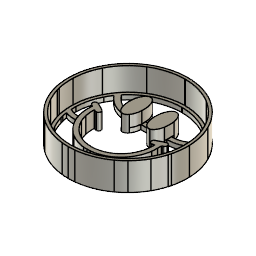
Smiley Face v5 (Autodesk Fusion 360 design; units mm, degrees)
Autodesk Fusion 360 part; units mm, degrees
(part 1 of 2)
sketch "Sketch4" plane through (0, 0, 0) normal (0, 0, 1) x (1, 0, 0)
  spline S0 degree 3 poles (22.3929, -49.7183) (18.1084, -49.2352) (14.0604, -47.6727) (10.6177, -45.1732) knots 0 0 0 0 1 1 1 1
  spline S1 degree 3 poles (10.6177, -45.1732) (9.3741, -44.2703) (8.777, -43.7559) (7.5724, -42.5496) knots 0 0 0 0 1 1 1 1
  spline S2 degree 3 poles (7.5724, -42.5496) (5.8834, -40.8584) (4.627, -39.2036) (3.4694, -37.1458) knots 0 0 0 0 1 1 1 1
  spline S3 degree 3 poles (3.4694, -37.1458) (2.6439, -35.6786) (1.7398, -33.529) (1.3502, -32.1074) knots 0 0 0 0 1 1 1 1
  spline S4 degree 3 poles (1.3502, -32.1074) (1.2509, -31.7452) (1.1157, -31.2562) (1.0497, -31.0207) knots 0 0 0 0 1 1 1 1
  spline S5 degree 3 poles (1.0497, -31.0207) (0.5782, -29.3376) (0.2735, -26.3861) (0.3562, -24.3029) knots 0 0 0 0 1 1 1 1
  spline S6 degree 3 poles (0.3562, -24.3029) (0.5048, -20.5588) (1.3013, -17.4096) (2.9297, -14.1273) knots 0 0 0 0 1 1 1 1
  spline S7 degree 3 poles (2.9297, -14.1273) (5.04, -9.8738) (7.9486, -6.665) (12.0751, -4.0377) knots 0 0 0 0 1 1 1 1
  spline S8 degree 3 poles (12.0751, -4.0377) (15.652, -1.7603) (20.598, -0.3264) (24.8627, -0.3305) knots 0 0 0 0 1 1 1 1
  spline S9 degree 3 poles (35.9401, -2.8345) (38.3777, -4.0025) (40.6839, -5.6448) (42.5585, -7.5475) knots 0 0 0 0 1 1 1 1
  spline S10 degree 3 poles (42.5585, -7.5475) (44.9078, -9.9319) (46.4936, -12.2272) (47.7162, -15.0126) knots 0 0 0 0 1 1 1 1
  spline S11 degree 3 poles (47.7162, -15.0126) (48.8453, -17.585) (49.42, -19.722) (49.727, -22.4897) knots 0 0 0 0 1 1 1 1
  spline S12 degree 3 poles (49.727, -22.4897) (49.8539, -23.634) (49.8685, -24.0363) (49.8392, -25.5852) knots 0 0 0 0 1 1 1 1
  spline S13 degree 3 poles (49.8392, -25.5852) (49.8185, -26.682) (49.764, -27.6688) (49.6973, -28.1558) knots 0 0 0 0 1 1 1 1
  spline S14 degree 3 poles (49.6973, -28.1558) (49.4235, -30.1555) (48.9497, -32.0707) (48.3189, -33.7273) knots 0 0 0 0 1 1 1 1
  spline S15 degree 3 poles (48.3189, -33.7273) (47.8422, -34.9792) (47.8271, -35.0136) (47.1957, -36.2827) knots 0 0 0 0 1 1 1 1
  spline S16 degree 3 poles (47.1957, -36.2827) (45.3368, -40.0194) (42.3135, -43.4265) (38.7924, -45.7527) knots 0 0 0 0 1 1 1 1
  spline S17 degree 3 poles (38.7924, -45.7527) (35.9102, -47.6569) (32.2897, -49.0659) (29.001, -49.5633) knots 0 0 0 0 1 1 1 1
  spline S18 degree 3 poles (28.2875, -48.3499) (30.1103, -48.0656) (31.6025, -47.7001) (32.9844, -47.1994) knots 0 0 0 0 1 1 1 1
  spline S19 degree 3 poles (32.9844, -47.1994) (35.4347, -46.3115) (37.685, -45.0566) (39.7803, -43.4096) knots 0 0 0 0 1 1 1 1
  spline S20 degree 3 poles (39.7803, -43.4096) (40.5871, -42.7755) (42.7723, -40.5902) (43.4202, -39.7698) knots 0 0 0 0 1 1 1 1
  spline S21 degree 3 poles (43.4202, -39.7698) (45.9946, -36.5096) (47.7291, -32.5341) (48.315, -28.5509) knots 0 0 0 0 1 1 1 1
  spline S22 degree 3 poles (48.315, -28.5509) (48.4563, -27.591) (48.4958, -27.0364) (48.5229, -25.636) knots 0 0 0 0 1 1 1 1
  spline S23 degree 3 poles (48.5229, -25.636) (48.5765, -22.8709) (48.3393, -20.9923) (47.627, -18.54) knots 0 0 0 0 1 1 1 1
  spline S24 degree 3 poles (47.627, -18.54) (46.3739, -14.2261) (43.988, -10.489) (40.5598, -7.4706) knots 0 0 0 0 1 1 1 1
  spline S25 degree 3 poles (40.5598, -7.4706) (37.4385, -4.7224) (33.6744, -2.8804) (29.473, -2.0449) knots 0 0 0 0 1 1 1 1
  spline S26 degree 3 poles (21.4837, -1.9176) (18.0502, -2.4796) (15.0363, -3.6458) (12.2651, -5.4846) knots 0 0 0 0 1 1 1 1
  spline S27 degree 3 poles (12.2651, -5.4846) (10.7803, -6.4698) (9.6872, -7.3601) (8.5291, -8.5273) knots 0 0 0 0 1 1 1 1
  spline S28 degree 3 poles (8.5291, -8.5273) (4.5448, -12.543) (2.2228, -17.5622) (1.7183, -23.2491) knots 0 0 0 0 1 1 1 1
  spline S29 degree 3 poles (1.7183, -23.2491) (1.5776, -24.8363) (1.6754, -27.2522) (1.945, -28.8466) knots 0 0 0 0 1 1 1 1
  spline S30 degree 3 poles (1.945, -28.8466) (3.4362, -37.665) (9.5432, -44.731) (18.046, -47.4762) knots 0 0 0 0 1 1 1 1
  spline S31 degree 3 poles (18.046, -47.4762) (19.4801, -47.9392) (21.486, -48.3368) (23.2161, -48.5011) knots 0 0 0 0 1 1 1 1
  spline S32 degree 3 poles (25.4554, -48.5048) (27.035, -48.4878) (27.603, -48.4567) (28.2875, -48.3499) knots 0 0 0 0 1 1 1 1
  spline S33 degree 3 poles (23.5455, -42.8964) (21.5099, -42.7183) (18.9093, -41.8162) (17.0581, -40.646) knots 0 0 0 0 1 1 1 1
  spline S34 degree 3 poles (17.0581, -40.646) (16.2134, -40.1121) (15.1136, -39.2029) (14.3454, -38.4035) knots 0 0 0 0 1 1 1 1
  spline S35 degree 3 poles (14.3454, -38.4035) (12.0712, -36.0367) (10.6196, -33.0647) (10.096, -29.7035) knots 0 0 0 0 1 1 1 1
  spline S36 degree 3 poles (10.096, -29.7035) (10.0046, -29.1166) (9.9786, -28.5661) (9.9809, -27.2582) knots 0 0 0 0 1 1 1 1
  line L0 (9.9809, -27.2582) -> (9.9837, -25.5702)
  line L1 (9.9837, -25.5702) -> (9.5685, -25.3593)
  spline S37 degree 3 poles (9.5685, -25.3593) (8.985, -25.0629) (8.7925, -24.7926) (8.7925, -24.2699) knots 0 0 0 0 1 1 1 1
  spline S38 degree 3 poles (8.7925, -24.2699) (8.7925, -23.9246) (8.8206, -23.8276) (8.9823, -23.6157) knots 0 0 0 0 1 1 1 1
  spline S39 degree 3 poles (8.9823, -23.6157) (9.0867, -23.4788) (9.271, -23.3255) (9.3918, -23.275) knots 0 0 0 0 1 1 1 1
  spline S40 degree 3 poles (9.3918, -23.275) (9.865, -23.0773) (10.0223, -23.1273) (11.92, -24.0791) knots 0 0 0 0 1 1 1 1
  spline S41 degree 3 poles (11.92, -24.0791) (13.4801, -24.8616) (13.727, -25.0063) (13.87, -25.2225) knots 0 0 0 0 1 1 1 1
  spline S42 degree 3 poles (13.87, -25.2225) (14.3541, -25.9539) (13.9374, -26.8519) (13.081, -26.923) knots 0 0 0 0 1 1 1 1
  spline S43 degree 3 poles (13.081, -26.923) (12.7923, -26.9469) (12.6703, -26.9186) (12.3363, -26.7499) knots 0 0 0 0 1 1 1 1
  spline S44 degree 3 poles (12.3363, -26.7499) (12.1165, -26.639) (11.9184, -26.5666) (11.8959, -26.5891) knots 0 0 0 0 1 1 1 1
  spline S45 degree 3 poles (11.8959, -26.5891) (11.7452, -26.7398) (11.9635, -29.5037) (12.2147, -30.6256) knots 0 0 0 0 1 1 1 1
  spline S46 degree 3 poles (12.2147, -30.6256) (12.3647, -31.2958) (12.9496, -32.9532) (13.2453, -33.5457) knots 0 0 0 0 1 1 1 1
  spline S47 degree 3 poles (13.2453, -33.5457) (14.0979, -35.2549) (15.1952, -36.6806) (16.5766, -37.8744) knots 0 0 0 0 1 1 1 1
  spline S48 degree 3 poles (26.9703, -40.8582) (28.8487, -40.5706) (30.9888, -39.6668) (32.5246, -38.5124) knots 0 0 0 0 1 1 1 1
  spline S49 degree 3 poles (32.5246, -38.5124) (35.3434, -36.3938) (37.2177, -33.2749) (37.8383, -29.6706) knots 0 0 0 0 1 1 1 1
  spline S50 degree 3 poles (37.8383, -29.6706) (37.9441, -29.0562) (38.0514, -26.8316) (37.9837, -26.6553) knots 0 0 0 0 1 1 1 1
  spline S51 degree 3 poles (37.9837, -26.6553) (37.9514, -26.5712) (37.8838, -26.5863) (37.562, -26.7497) knots 0 0 0 0 1 1 1 1
  spline S52 degree 3 poles (37.562, -26.7497) (36.6703, -27.2024) (35.7932, -26.7484) (35.8056, -25.8403) knots 0 0 0 0 1 1 1 1
  spline S53 degree 3 poles (35.8056, -25.8403) (35.8109, -25.4521) (35.9816, -25.1239) (36.2701, -24.9477) knots 0 0 0 0 1 1 1 1
  spline S54 degree 3 poles (36.2701, -24.9477) (36.3714, -24.8858) (37.1903, -24.4635) (38.0899, -24.0092) knots 0 0 0 0 1 1 1 1
  spline S55 degree 3 poles (38.0899, -24.0092) (39.8842, -23.1031) (40.0208, -23.0647) (40.5459, -23.3189) knots 0 0 0 0 1 1 1 1
  spline S56 degree 3 poles (40.5459, -23.3189) (40.9989, -23.5382) (41.2211, -24.1649) (41.0275, -24.6773) knots 0 0 0 0 1 1 1 1
  spline S57 degree 3 poles (41.0275, -24.6773) (40.9219, -24.9567) (40.6754, -25.1821) (40.2565, -25.3823) knots 0 0 0 0 1 1 1 1
  line L2 (40.2565, -25.3823) -> (39.8791, -25.5627)
  line L3 (39.8791, -25.5627) -> (39.8761, -27.3532)
  spline S58 degree 3 poles (39.8761, -27.3532) (39.8729, -29.2446) (39.794, -29.9764) (39.4487, -31.3197) knots 0 0 0 0 1 1 1 1
  spline S59 degree 3 poles (39.4487, -31.3197) (38.8984, -33.4603) (37.6825, -35.9163) (36.4341, -37.4093) knots 0 0 0 0 1 1 1 1
  spline S60 degree 3 poles (36.4341, -37.4093) (35.9443, -37.9949) (34.8466, -39.1017) (34.3138, -39.5469) knots 0 0 0 0 1 1 1 1
  spline S61 degree 3 poles (34.3138, -39.5469) (32.1741, -41.3351) (29.3055, -42.5474) (26.4434, -42.8731) knots 0 0 0 0 1 1 1 1
  spline S62 degree 3 poles (18.8364, -21.7662) (17.7438, -21.4052) (16.831, -19.9501) (16.3899, -17.8664) knots 0 0 0 0 1 1 1 1
  spline S63 degree 3 poles (16.3899, -17.8664) (16.1877, -16.9113) (16.1678, -14.6605) (16.3533, -13.7321) knots 0 0 0 0 1 1 1 1
  spline S64 degree 3 poles (16.3533, -13.7321) (16.7289, -11.8523) (17.4711, -10.4695) (18.4214, -9.8792) knots 0 0 0 0 1 1 1 1
  spline S65 degree 3 poles (18.4214, -9.8792) (18.7703, -9.6625) (18.8263, -9.6487) (19.3578, -9.6487) knots 0 0 0 0 1 1 1 1
  spline S66 degree 3 poles (19.3578, -9.6487) (19.8618, -9.6487) (19.958, -9.6692) (20.2453, -9.8381) knots 0 0 0 0 1 1 1 1
  spline S67 degree 3 poles (20.2453, -9.8381) (21.7561, -10.7261) (22.7124, -13.6271) (22.4687, -16.5828) knots 0 0 0 0 1 1 1 1
  spline S68 degree 3 poles (22.4687, -16.5828) (22.3227, -18.3534) (21.936, -19.6054) (21.1995, -20.6915) knots 0 0 0 0 1 1 1 1
  spline S69 degree 3 poles (21.1995, -20.6915) (20.5927, -21.5865) (19.6247, -22.0267) (18.8364, -21.7662) knots 0 0 0 0 1 1 1 1
  spline S70 degree 3 poles (30.3292, -21.8073) (29.1191, -21.4923) (28.1324, -19.933) (27.7198, -17.6838) knots 0 0 0 0 1 1 1 1
  spline S71 degree 3 poles (27.7198, -17.6838) (27.5511, -16.7641) (27.5165, -15.0092) (27.6496, -14.1273) knots 0 0 0 0 1 1 1 1
  spline S72 degree 3 poles (27.6496, -14.1273) (27.9104, -12.4) (28.5146, -10.9962) (29.3283, -10.2266) knots 0 0 0 0 1 1 1 1
  spline S73 degree 3 poles (29.3283, -10.2266) (29.7997, -9.7808) (30.0439, -9.6661) (30.5981, -9.6301) knots 0 0 0 0 1 1 1 1
  spline S74 degree 3 poles (30.5981, -9.6301) (30.9744, -9.6057) (31.125, -9.6266) (31.3772, -9.7381) knots 0 0 0 0 1 1 1 1
  spline S75 degree 3 poles (31.3772, -9.7381) (31.7947, -9.9228) (32.1305, -10.197) (32.4561, -10.6191) knots 0 0 0 0 1 1 1 1
  spline S76 degree 3 poles (32.4561, -10.6191) (34.1715, -12.8426) (34.3373, -17.698) (32.788, -20.3387) knots 0 0 0 0 1 1 1 1
  spline S77 degree 3 poles (32.788, -20.3387) (32.4993, -20.8307) (31.8262, -21.5083) (31.4696, -21.6659) knots 0 0 0 0 1 1 1 1
  spline S78 degree 3 poles (31.4696, -21.6659) (31.134, -21.8141) (30.6066, -21.8796) (30.3292, -21.8073) knots 0 0 0 0 1 1 1 1
  line L4 (25, -0.2) -> (25, -49.8487) construction
  spline S79 degree 3 poles (29.473, -2.0449) (28.1481, -1.7814) (26.5625, -1.6493) (25, -1.6529) knots 0 0 0 0 0.55892 0.55892 0.55892 0.55892
  spline S80 degree 3 poles (25, -1.6529) (23.7669, -1.6558) (22.5483, -1.7433) (21.4837, -1.9176) knots 0.55892 0.55892 0.55892 0.55892 1 1 1 1
  spline S81 degree 3 poles (16.5766, -37.8744) (18.9879, -39.9581) (21.902, -41.0359) (25, -41.0162) knots 0 0 0 0 0.826651 0.826651 0.826651 0.826651
  spline S82 degree 3 poles (25, -41.0162) (25.6496, -41.0121) (26.3074, -40.9597) (26.9703, -40.8582) knots 0.826651 0.826651 0.826651 0.826651 1 1 1 1
  spline S83 degree 3 poles (26.4434, -42.8731) (26.1661, -42.9047) (25.5854, -42.9239) (25, -42.9283) knots 0 0 0 0 0.504698 0.504698 0.504698 0.504698
  spline S84 degree 3 poles (25, -42.9283) (24.4255, -42.9327) (23.8466, -42.9228) (23.5455, -42.8964) knots 0.504698 0.504698 0.504698 0.504698 1 1 1 1
  spline S85 degree 3 poles (23.2161, -48.5011) (23.3405, -48.5129) (24.1002, -48.5158) (25, -48.509) knots 0 0 0 0 0.858151 0.858151 0.858151 0.858151
  spline S86 degree 3 poles (25, -48.509) (25.1487, -48.5078) (25.3013, -48.5064) (25.4554, -48.5048) knots 0.858151 0.858151 0.858151 0.858151 1 1 1 1
  spline S87 degree 3 poles (29.001, -49.5633) (27.7693, -49.7496) (26.3539, -49.8467) (25, -49.8487) knots 0 0 0 0 0.594454 0.594454 0.594454 0.594454
  spline S88 degree 3 poles (25, -49.8487) (24.0764, -49.8501) (23.1814, -49.8072) (22.3929, -49.7183) knots 0.594454 0.594454 0.594454 0.594454 1 1 1 1
  spline S89 degree 3 poles (24.8627, -0.3305) (24.9085, -0.3305) (24.9543, -0.3307) (25, -0.3309) knots 0 0 0 0 0.011443 0.011443 0.011443 0.011443
  spline S90 degree 3 poles (25, -0.3309) (28.9486, -0.3525) (32.4187, -1.1472) (35.9401, -2.8345) knots 0.011443 0.011443 0.011443 0.011443 1 1 1 1
  constraint vertical L4
  constraint coincident L4 S79.end
  constraint coincident L4 S81.end
  constraint coincident L4 S83.end
  constraint coincident L4 S85.end
  constraint coincident L4 S89.end
sketch "Sketch5" plane through (0, 0, 0) normal (0, 0, 1) x (1, 0, 0)
  spline S0 degree 3 poles (24.8627, -0.3305) (24.9085, -0.3305) (24.9543, -0.3307) (25, -0.3309) knots 0 0 0 0 0.011443 0.011443 0.011443 0.011443
  spline S1 degree 3 poles (12.0751, -4.0377) (15.652, -1.7603) (20.598, -0.3264) (24.8627, -0.3305) knots 0 0 0 0 1 1 1 1
  spline S2 degree 3 poles (2.9297, -14.1273) (5.04, -9.8738) (7.9486, -6.665) (12.0751, -4.0377) knots 0 0 0 0 1 1 1 1
  spline S3 degree 3 poles (0.3562, -24.3029) (0.5048, -20.5588) (1.3013, -17.4096) (2.9297, -14.1273) knots 0 0 0 0 1 1 1 1
  spline S4 degree 3 poles (1.0497, -31.0207) (0.5782, -29.3376) (0.2735, -26.3861) (0.3562, -24.3029) knots 0 0 0 0 1 1 1 1
  spline S5 degree 3 poles (3.4694, -37.1458) (2.6439, -35.6786) (1.7398, -33.529) (1.3502, -32.1074) knots 0 0 0 0 1 1 1 1
  spline S6 degree 3 poles (1.3502, -32.1074) (1.2509, -31.7452) (1.1157, -31.2562) (1.0497, -31.0207) knots 0 0 0 0 1 1 1 1
  spline S7 degree 3 poles (7.5724, -42.5496) (5.8834, -40.8584) (4.627, -39.2036) (3.4694, -37.1458) knots 0 0 0 0 1 1 1 1
  spline S8 degree 3 poles (10.6177, -45.1732) (9.3741, -44.2703) (8.777, -43.7559) (7.5724, -42.5496) knots 0 0 0 0 1 1 1 1
  spline S9 degree 3 poles (22.3929, -49.7183) (18.1084, -49.2352) (14.0604, -47.6727) (10.6177, -45.1732) knots 0 0 0 0 1 1 1 1
  spline S10 degree 3 poles (25, -49.8487) (24.0764, -49.8501) (23.1814, -49.8072) (22.3929, -49.7183) knots 0.594454 0.594454 0.594454 0.594454 1 1 1 1
  spline S11 degree 3 poles (25, -42.9283) (24.4255, -42.9327) (23.8466, -42.9228) (23.5455, -42.8964) knots 0.504698 0.504698 0.504698 0.504698 1 1 1 1
  spline S12 degree 3 poles (23.5455, -42.8964) (21.5099, -42.7183) (18.9093, -41.8162) (17.0581, -40.646) knots 0 0 0 0 1 1 1 1
  spline S13 degree 3 poles (17.0581, -40.646) (16.2134, -40.1121) (15.1136, -39.2029) (14.3454, -38.4035) knots 0 0 0 0 1 1 1 1
  spline S14 degree 3 poles (14.3454, -38.4035) (12.0712, -36.0367) (10.6196, -33.0647) (10.096, -29.7035) knots 0 0 0 0 1 1 1 1
  spline S15 degree 3 poles (10.096, -29.7035) (10.0046, -29.1166) (9.9786, -28.5661) (9.9809, -27.2582) knots 0 0 0 0 1 1 1 1
  line L0 (9.9809, -27.2582) -> (9.9837, -25.5702)
  line L1 (9.9837, -25.5702) -> (9.5685, -25.3593)
  spline S16 degree 3 poles (9.5685, -25.3593) (8.985, -25.0629) (8.7925, -24.7926) (8.7925, -24.2699) knots 0 0 0 0 1 1 1 1
  spline S17 degree 3 poles (8.7925, -24.2699) (8.7925, -23.9246) (8.8206, -23.8276) (8.9823, -23.6157) knots 0 0 0 0 1 1 1 1
  spline S18 degree 3 poles (8.9823, -23.6157) (9.0867, -23.4788) (9.271, -23.3255) (9.3918, -23.275) knots 0 0 0 0 1 1 1 1
  spline S19 degree 3 poles (9.3918, -23.275) (9.865, -23.0773) (10.0223, -23.1273) (11.92, -24.0791) knots 0 0 0 0 1 1 1 1
  spline S20 degree 3 poles (11.92, -24.0791) (13.4801, -24.8616) (13.727, -25.0063) (13.87, -25.2225) knots 0 0 0 0 1 1 1 1
  spline S21 degree 3 poles (13.87, -25.2225) (14.3541, -25.9539) (13.9374, -26.8519) (13.081, -26.923) knots 0 0 0 0 1 1 1 1
  spline S22 degree 3 poles (13.081, -26.923) (12.7923, -26.9469) (12.6703, -26.9186) (12.3363, -26.7499) knots 0 0 0 0 1 1 1 1
  spline S23 degree 3 poles (12.3363, -26.7499) (12.1165, -26.639) (11.9184, -26.5666) (11.8959, -26.5891) knots 0 0 0 0 1 1 1 1
  spline S24 degree 3 poles (11.8959, -26.5891) (11.7452, -26.7398) (11.9635, -29.5037) (12.2147, -30.6256) knots 0 0 0 0 1 1 1 1
  spline S25 degree 3 poles (12.2147, -30.6256) (12.3647, -31.2958) (12.9496, -32.9532) (13.2453, -33.5457) knots 0 0 0 0 1 1 1 1
  spline S26 degree 3 poles (13.2453, -33.5457) (14.0979, -35.2549) (15.1952, -36.6806) (16.5766, -37.8744) knots 0 0 0 0 1 1 1 1
  spline S27 degree 3 poles (16.5766, -37.8744) (18.9879, -39.9581) (21.902, -41.0359) (25, -41.0162) knots 0 0 0 0 0.826651 0.826651 0.826651 0.826651
  spline S28 degree 3 poles (18.8364, -21.7662) (17.7438, -21.4052) (16.831, -19.9501) (16.3899, -17.8664) knots 0 0 0 0 1 1 1 1
  spline S29 degree 3 poles (16.3899, -17.8664) (16.1877, -16.9113) (16.1678, -14.6605) (16.3533, -13.7321) knots 0 0 0 0 1 1 1 1
  spline S30 degree 3 poles (16.3533, -13.7321) (16.7289, -11.8523) (17.4711, -10.4695) (18.4214, -9.8792) knots 0 0 0 0 1 1 1 1
  spline S31 degree 3 poles (18.4214, -9.8792) (18.7703, -9.6625) (18.8263, -9.6487) (19.3578, -9.6487) knots 0 0 0 0 1 1 1 1
  spline S32 degree 3 poles (19.3578, -9.6487) (19.8618, -9.6487) (19.958, -9.6692) (20.2453, -9.8381) knots 0 0 0 0 1 1 1 1
  spline S33 degree 3 poles (20.2453, -9.8381) (21.7561, -10.7261) (22.7124, -13.6271) (22.4687, -16.5828) knots 0 0 0 0 1 1 1 1
  spline S34 degree 3 poles (21.1995, -20.6915) (20.5927, -21.5865) (19.6247, -22.0267) (18.8364, -21.7662) knots 0 0 0 0 1 1 1 1
  spline S35 degree 3 poles (22.4687, -16.5828) (22.3227, -18.3534) (21.936, -19.6054) (21.1995, -20.6915) knots 0 0 0 0 1 1 1 1
  line L2 (25, -0.3309) -> (25, -49.8487) construction
  spline S36 degree 3 poles (25, -49.8487) (25.9236, -49.8501) (26.8186, -49.8072) (27.6071, -49.7183) knots 0.594454 0.594454 0.594454 0.594454 1 1 1 1
  spline S37 degree 3 poles (27.6071, -49.7183) (31.8916, -49.2352) (35.9396, -47.6727) (39.3823, -45.1732) knots 0 0 0 0 1 1 1 1
  spline S38 degree 3 poles (39.3823, -45.1732) (40.6259, -44.2703) (41.223, -43.7559) (42.4276, -42.5496) knots 0 0 0 0 1 1 1 1
  spline S39 degree 3 poles (42.4276, -42.5496) (44.1166, -40.8584) (45.373, -39.2036) (46.5306, -37.1458) knots 0 0 0 0 1 1 1 1
  spline S40 degree 3 poles (46.5306, -37.1458) (47.3561, -35.6786) (48.2602, -33.529) (48.6498, -32.1074) knots 0 0 0 0 1 1 1 1
  spline S41 degree 3 poles (48.6498, -32.1074) (48.7491, -31.7452) (48.8843, -31.2562) (48.9503, -31.0207) knots 0 0 0 0 1 1 1 1
  spline S42 degree 3 poles (48.9503, -31.0207) (49.4218, -29.3376) (49.7265, -26.3861) (49.6438, -24.3029) knots 0 0 0 0 1 1 1 1
  spline S43 degree 3 poles (49.6438, -24.3029) (49.4952, -20.5588) (48.6987, -17.4096) (47.0703, -14.1273) knots 0 0 0 0 1 1 1 1
  spline S44 degree 3 poles (47.0703, -14.1273) (44.96, -9.8738) (42.0514, -6.665) (37.9249, -4.0377) knots 0 0 0 0 1 1 1 1
  spline S45 degree 3 poles (25.1373, -0.3305) (25.0915, -0.3305) (25.0457, -0.3307) (25, -0.3309) knots 0 0 0 0 0.011443 0.011443 0.011443 0.011443
  spline S46 degree 3 poles (37.9249, -4.0377) (34.348, -1.7603) (29.402, -0.3264) (25.1373, -0.3305) knots 0 0 0 0 1 1 1 1
  spline S47 degree 3 poles (30.6422, -9.6487) (30.1382, -9.6487) (30.042, -9.6692) (29.7547, -9.8381) knots 0 0 0 0 1 1 1 1
  spline S48 degree 3 poles (29.7547, -9.8381) (28.2439, -10.7261) (27.2876, -13.6271) (27.5313, -16.5828) knots 0 0 0 0 1 1 1 1
  spline S49 degree 3 poles (27.5313, -16.5828) (27.6773, -18.3534) (28.064, -19.6054) (28.8005, -20.6915) knots 0 0 0 0 1 1 1 1
  spline S50 degree 3 poles (28.8005, -20.6915) (29.4073, -21.5865) (30.3753, -22.0267) (31.1636, -21.7662) knots 0 0 0 0 1 1 1 1
  spline S51 degree 3 poles (31.1636, -21.7662) (32.2562, -21.4052) (33.169, -19.9501) (33.6101, -17.8664) knots 0 0 0 0 1 1 1 1
  spline S52 degree 3 poles (33.6101, -17.8664) (33.8123, -16.9113) (33.8322, -14.6605) (33.6467, -13.7321) knots 0 0 0 0 1 1 1 1
  spline S53 degree 3 poles (31.5786, -9.8792) (31.2297, -9.6625) (31.1737, -9.6487) (30.6422, -9.6487) knots 0 0 0 0 1 1 1 1
  spline S54 degree 3 poles (33.6467, -13.7321) (33.2711, -11.8523) (32.5289, -10.4695) (31.5786, -9.8792) knots 0 0 0 0 1 1 1 1
  spline S55 degree 3 poles (25, -42.9283) (25.5745, -42.9327) (26.1534, -42.9228) (26.4545, -42.8964) knots 0.504698 0.504698 0.504698 0.504698 1 1 1 1
  spline S56 degree 3 poles (26.4545, -42.8964) (28.4901, -42.7183) (31.0907, -41.8162) (32.9419, -40.646) knots 0 0 0 0 1 1 1 1
  spline S57 degree 3 poles (32.9419, -40.646) (33.7866, -40.1121) (34.8864, -39.2029) (35.6546, -38.4035) knots 0 0 0 0 1 1 1 1
  spline S58 degree 3 poles (35.6546, -38.4035) (37.9288, -36.0367) (39.3804, -33.0647) (39.904, -29.7035) knots 0 0 0 0 1 1 1 1
  spline S59 degree 3 poles (39.904, -29.7035) (39.9954, -29.1166) (40.0214, -28.5661) (40.0191, -27.2582) knots 0 0 0 0 1 1 1 1
  line L3 (40.0191, -27.2582) -> (40.0163, -25.5702)
  line L4 (40.0163, -25.5702) -> (40.4315, -25.3593)
  spline S60 degree 3 poles (40.4315, -25.3593) (41.015, -25.0629) (41.2075, -24.7926) (41.2075, -24.2699) knots 0 0 0 0 1 1 1 1
  spline S61 degree 3 poles (41.2075, -24.2699) (41.2075, -23.9246) (41.1794, -23.8276) (41.0177, -23.6157) knots 0 0 0 0 1 1 1 1
  spline S62 degree 3 poles (41.0177, -23.6157) (40.9133, -23.4788) (40.729, -23.3255) (40.6082, -23.275) knots 0 0 0 0 1 1 1 1
  spline S63 degree 3 poles (38.08, -24.0791) (36.5199, -24.8616) (36.273, -25.0063) (36.13, -25.2225) knots 0 0 0 0 1 1 1 1
  spline S64 degree 3 poles (36.13, -25.2225) (35.6459, -25.9539) (36.0626, -26.8519) (36.919, -26.923) knots 0 0 0 0 1 1 1 1
  spline S65 degree 3 poles (36.919, -26.923) (37.2077, -26.9469) (37.3297, -26.9186) (37.6637, -26.7499) knots 0 0 0 0 1 1 1 1
  spline S66 degree 3 poles (37.6637, -26.7499) (37.8835, -26.639) (38.0816, -26.5666) (38.1041, -26.5891) knots 0 0 0 0 1 1 1 1
  spline S67 degree 3 poles (38.1041, -26.5891) (38.2548, -26.7398) (38.0365, -29.5037) (37.7853, -30.6256) knots 0 0 0 0 1 1 1 1
  spline S68 degree 3 poles (37.7853, -30.6256) (37.6353, -31.2958) (37.0504, -32.9532) (36.7547, -33.5457) knots 0 0 0 0 1 1 1 1
  spline S69 degree 3 poles (36.7547, -33.5457) (35.9021, -35.2549) (34.8048, -36.6806) (33.4234, -37.8744) knots 0 0 0 0 1 1 1 1
  spline S70 degree 3 poles (33.4234, -37.8744) (31.0121, -39.9581) (28.098, -41.0359) (25, -41.0162) knots 0 0 0 0 0.826651 0.826651 0.826651 0.826651
  spline S71 degree 3 poles (40.6082, -23.275) (40.135, -23.0773) (39.9777, -23.1273) (38.08, -24.0791) knots 0 0 0 0 1 1 1 1
  spline S72 degree 3 poles (25.1362, 0.8695) (25.0907, 0.8695) (25.0453, 0.8693) (25, 0.8691) knots 0 0 0 0 0.010916 0.010916 0.010916 0.010916
  spline S73 degree 3 poles (24.8638, 0.8695) (24.9093, 0.8695) (24.9547, 0.8693) (25, 0.8691) knots 0 0 0 0 0.010916 0.010916 0.010916 0.010916
  spline S74 degree 3 poles (11.4307, -3.0254) (15.2378, -0.6015) (20.3293, 0.8738) (24.8638, 0.8695) knots 0 0 0 0 1 1 1 1
  spline S75 degree 3 poles (1.8548, -13.5939) (4.0534, -9.1625) (7.1462, -5.7533) (11.4307, -3.0254) knots 0 0 0 0 1 1 1 1
  spline S76 degree 3 poles (-0.8429, -24.2553) (-0.6886, -20.3681) (0.1597, -17.0105) (1.8548, -13.5939) knots 0 0 0 0 1 1 1 1
  spline S77 degree 3 poles (-0.1058, -31.3445) (-0.5059, -29.9163) (-0.7593, -27.9125) (-0.8356, -26.045) (-0.861, -25.4219) (-0.8652, -24.8169) (-0.8429, -24.2553) knots 0 0 0 0 0.749811 0.749811 0.749811 1 1 1 1
  spline S78 degree 3 poles (0.1929, -32.4246) (0.0942, -32.0647) (-0.0413, -31.5745) (-0.1058, -31.3445) knots 0 0 0 0 0.999998 0.999998 0.999998 0.999998
  spline S79 degree 3 poles (2.4235, -37.7342) (1.5361, -36.1568) (0.6261, -34.0052) (0.1929, -32.4246) knots 0 0 0 0 1 1 1 1
  spline S80 degree 3 poles (6.7233, -43.3976) (4.968, -41.64) (3.6282, -39.8758) (2.4235, -37.7342) knots 0 0 0 0 1 1 1 1
  spline S81 degree 3 poles (9.9127, -46.1443) (8.6415, -45.2214) (7.9474, -44.6234) (6.7233, -43.3976) knots 0 0 0 0 1 1 1 1
  spline S82 degree 3 poles (22.2584, -50.9107) (17.7713, -50.4048) (13.5248, -48.7669) (9.9127, -46.1443) knots 0 0 0 0 1 1 1 1
  spline S83 degree 3 poles (24.9982, -51.0487) (24.0376, -51.05) (23.1037, -51.006) (22.2584, -50.9107) knots 0.594956 0.594956 0.594956 0.594956 1 1 1 1
  spline S84 degree 3 poles (24.9982, -51.0487) (25.9601, -51.0501) (26.8953, -51.0062) (27.7416, -50.9107) knots 0.594454 0.594454 0.594454 0.594454 1 1 1 1
  spline S85 degree 3 poles (27.7416, -50.9107) (32.2287, -50.4048) (36.4752, -48.7669) (40.0873, -46.1443) knots 0 0 0 0 1 1 1 1
  spline S86 degree 3 poles (40.0873, -46.1443) (41.3585, -45.2214) (42.0526, -44.6234) (43.2767, -43.3976) knots 0 0 0 0 1 1 1 1
  spline S87 degree 3 poles (43.2767, -43.3976) (45.032, -41.64) (46.3718, -39.8758) (47.5765, -37.7342) knots 0 0 0 0 1 1 1 1
  spline S88 degree 3 poles (47.5765, -37.7342) (48.4639, -36.1568) (49.3739, -34.0052) (49.8071, -32.4246) knots 0 0 0 0 1 1 1 1
  spline S89 degree 3 poles (49.8071, -32.4246) (49.9058, -32.0647) (50.0413, -31.5744) (50.1058, -31.3445) knots 0 0 0 0 1 1 1 1
  spline S90 degree 3 poles (50.1058, -31.3445) (50.5059, -29.9163) (50.7593, -27.9125) (50.8356, -26.045) (50.861, -25.4219) (50.8652, -24.8169) (50.8429, -24.2553) knots 0 0 0 0 0.749811 0.749811 0.749811 1 1 1 1
  spline S91 degree 3 poles (50.8429, -24.2553) (50.6886, -20.3681) (49.8403, -17.0105) (48.1452, -13.5939) knots 0 0 0 0 1 1 1 1
  spline S92 degree 3 poles (48.1452, -13.5939) (45.9466, -9.1625) (42.8538, -5.7533) (38.5693, -3.0254) knots 0 0 0 0 1 1 1 1
  spline S93 degree 3 poles (38.5693, -3.0254) (34.7622, -0.6015) (29.6707, 0.8738) (25.1362, 0.8695) knots 0 0 0 0 1 1 1 1
  spline S94 degree 5 poles (6.2927, -8.9882) (6.7312, -9.5928) (7.5942, -10.7006) (8.8467, -12.0587) (10.4463, -13.3414) (12.3816, -14.3288) (13.919, -14.7717) (15.0833, -14.9392) (15.8671, -14.9765) (16.2609, -14.9765) knots 0 0 0 0 0 0 0.2 0.4 0.6 0.8 1 1 1 1 1 1
  line L5 (5.2421, -7.5397) -> (7.3433, -10.4366)
  line L6 (15.3452, -14.9765) -> (17.1765, -14.9765)
  spline S95 degree 3 poles (4.6947, -10.6517) (6.4227, -13.0275) (8.1945, -14.5562) (9.9453, -15.4812) (11.7704, -16.4456) (13.5129, -16.8223) (15.223, -16.9413) (15.5676, -16.9653) (15.9117, -16.9769) (16.2555, -16.9765) (16.262, -16.9765) (16.2685, -16.9765) (16.275, -16.9765) knots 0 0 0 0 0.443948 0.443948 0.443948 0.906729 0.906729 0.906729 1 1 1 1.00195 1.00195 1.00195 1.00195
  line L7 (22.4858, -14.9765) -> (27.5142, -14.9765)
  line L8 (22.4313, -16.9765) -> (27.5687, -16.9765)
  line L9 (24, -42.9197) -> (24, -49.8323)
  line L10 (26, -42.9197) -> (26, -49.8323)
  spline S96 degree 5 poles (0.3495, -25.5702) (0.8642, -25.9274) (1.8614, -26.5452) (3.261, -27.1829) (4.9563, -27.5281) (6.8533, -27.3542) (8.214, -26.8513) (9.1392, -26.2868) (9.7099, -25.8236) (9.9837, -25.5702) knots 0 0 0 0 0 0 0.2 0.4 0.6 0.8 1 1 1 1 1 1
  line L11 (-0.8555, -24.7341) -> (1.5545, -26.4064)
  line L12 (9.3674, -26.1404) -> (10.6, -25)
  spline S97 degree 3 poles (-0.7907, -27.2134) (1.2201, -28.6087) (3.1804, -29.3002) (4.9777, -29.384) (6.9564, -29.4763) (8.7014, -28.9281) (10.1956, -27.9395) (10.5986, -27.6729) (10.9821, -27.3712) (11.342, -27.0382) knots 0 0 0 0 0.417024 0.417024 0.417024 0.876153 0.876153 0.876153 1 1 1 1
  spline S98 degree 5 poles (43.7073, -8.9882) (43.2688, -9.5928) (42.4058, -10.7006) (41.1533, -12.0587) (39.5537, -13.3414) (37.6184, -14.3288) (36.081, -14.7717) (34.9167, -14.9392) (34.1329, -14.9765) (33.7391, -14.9765) knots 0 0 0 0 0 0 0.2 0.4 0.6 0.8 1 1 1 1 1 1
  line L13 (44.7579, -7.5397) -> (42.6567, -10.4366)
  line L14 (34.6548, -14.9765) -> (32.8235, -14.9765)
  spline S99 degree 3 poles (45.3053, -10.6517) (43.5773, -13.0275) (41.8055, -14.5562) (40.0547, -15.4812) (38.2296, -16.4456) (36.4871, -16.8223) (34.777, -16.9413) (34.4324, -16.9653) (34.0883, -16.9769) (33.7445, -16.9765) (33.738, -16.9765) (33.7315, -16.9765) (33.725, -16.9765) knots 0 0 0 0 0.443948 0.443948 0.443948 0.906729 0.906729 0.906729 1 1 1 1.00195 1.00195 1.00195 1.00195
  spline S100 degree 5 poles (49.6505, -25.5702) (49.1358, -25.9274) (48.1386, -26.5452) (46.739, -27.1829) (45.0437, -27.5281) (43.1467, -27.3542) (41.786, -26.8513) (40.8608, -26.2868) (40.2901, -25.8236) (40.0163, -25.5702) knots 0 0 0 0 0 0 0.2 0.4 0.6 0.8 1 1 1 1 1 1
  line L15 (50.8555, -24.7341) -> (48.4455, -26.4064)
  line L16 (40.6326, -26.1404) -> (39.4, -25)
  spline S101 degree 3 poles (50.7907, -27.2134) (48.7799, -28.6087) (46.8196, -29.3002) (45.0223, -29.384) (43.0436, -29.4763) (41.2986, -28.9281) (39.8044, -27.9395) (39.4014, -27.6729) (39.0179, -27.3712) (38.658, -27.0382) knots 0 0 0 0 0.417024 0.417024 0.417024 0.876153 0.876153 0.876153 1 1 1 1
  dimension "d9" = 1.2
  dimension "d11" = 2
  dimension "d12" = 2
  dimension "d13" = 2
  constraint coincident S0.end L2.start
  constraint coincident S10.start L2.end
  constraint symmetric S0.start L2 S45.start
  constraint symmetric S0.end L2 S45.end
  constraint symmetric S0 L2 S45
  constraint symmetric S1.start L2 S44.end
  constraint symmetric S1 L2 S46
  constraint symmetric S2.start L2 S43.end
  constraint symmetric S2 L2 S44
  constraint symmetric S3.start L2 S42.end
  constraint symmetric S3 L2 S43
  constraint symmetric S4.start L2 S41.end
  constraint symmetric S4 L2 S42
  constraint symmetric S5.start L2 S39.end
  constraint symmetric S5.end L2 S40.end
  constraint symmetric S5 L2 S40
  constraint symmetric S6 L2 S41
  constraint symmetric S7.start L2 S38.end
  constraint symmetric S7 L2 S39
  constraint symmetric S8.start L2 S37.end
  constraint symmetric S8 L2 S38
  constraint symmetric S9.start L2 S36.end
  constraint symmetric S9 L2 S37
  constraint symmetric S10.start L2 S36.start
  constraint symmetric S10 L2 S36
  constraint symmetric S11.start L2 S55.start
  constraint symmetric S11.end L2 S55.end
  constraint symmetric S11 L2 S55
  constraint symmetric S12.end L2 S56.end
  constraint symmetric S12 L2 S56
  constraint symmetric S13.end L2 S57.end
  constraint symmetric S13 L2 S57
  constraint symmetric S14.end L2 S58.end
  constraint symmetric S14 L2 S58
  constraint symmetric S15.end L2 S59.end
  constraint symmetric S15 L2 S59
  constraint symmetric L0.end L2 L3.end
  constraint symmetric L1.end L2 L4.end
  constraint symmetric S16.end L2 S60.end
  constraint symmetric S16 L2 S60
  constraint symmetric S17.end L2 S61.end
  constraint symmetric S17 L2 S61
  constraint symmetric S18.end L2 S62.end
  constraint symmetric S18 L2 S62
  constraint symmetric S19.end L2 S63.start
  constraint symmetric S19 L2 S71
  constraint symmetric S20.end L2 S63.end
  constraint symmetric S20 L2 S63
  constraint symmetric S21.end L2 S64.end
  constraint symmetric S21 L2 S64
  constraint symmetric S22.end L2 S65.end
  constraint symmetric S22 L2 S65
  constraint symmetric S23.end L2 S66.end
  constraint symmetric S23 L2 S66
  constraint symmetric S24.end L2 S67.end
  constraint symmetric S24 L2 S67
  constraint symmetric S25.end L2 S68.end
  constraint symmetric S25 L2 S68
  constraint symmetric S26.end L2 S69.end
  constraint symmetric S26 L2 S69
  constraint symmetric S27.end L2 S70.end
  constraint symmetric S27 L2 S70
  constraint symmetric S28.start L2 S50.end
  constraint symmetric S28.end L2 S51.end
  constraint symmetric S28 L2 S51
  constraint symmetric S29.end L2 S52.end
  constraint symmetric S29 L2 S52
  constraint symmetric S30.end L2 S53.start
  constraint symmetric S30 L2 S54
  constraint symmetric S31.end L2 S47.start
  constraint symmetric S31 L2 S53
  constraint symmetric S32.end L2 S47.end
  constraint symmetric S32 L2 S47
  constraint symmetric S33.end L2 S48.end
  constraint symmetric S33 L2 S48
  constraint symmetric S34.start L2 S49.end
  constraint symmetric S34 L2 S50
  constraint symmetric S35 L2 S49
  constraint coincident S2 S94.start
  constraint midpoint S94.start L5
  constraint midpoint S94.end L6
  constraint horizontal L6
  constraint coincident S29 S95.end
  constraint coincident S33 L7.start
  constraint coincident S48 L7.end
  constraint horizontal L7
  constraint coincident S35 L8.start
  constraint coincident S49 L8.end
  constraint parallel L7 L8
  constraint horizontal S95.end L8.start
  constraint horizontal S94.end L7.start
  constraint coincident S11 L9.start
  constraint coincident S10 L9.end
  constraint parallel L2 L9
  constraint coincident S36 L10.end
  constraint parallel L9 L10
  constraint symmetric L2 L9 L10
  constraint coincident S55 L10.start
  constraint coincident S4 S96.start
  constraint coincident L0.end L1.start
  constraint horizontal S96.start L0.end
  constraint midpoint S96.start L11
  constraint coincident S77 L11.start
  constraint midpoint L0.end L12
  constraint symmetric L2 S94.start S98.start
  constraint symmetric L2 S94.end S98.end
  constraint symmetric L2 L5.start L13.start
  constraint symmetric L2 L5.end L13.end
  constraint symmetric L2 L6.start L14.start
  constraint symmetric L2 L6.end L14.end
  constraint symmetric L2 S95.start S99.start
  constraint symmetric L2 S95.end S99.end
  constraint symmetric L2 S95 S99
  constraint symmetric L2 S96.start S100.start
  constraint symmetric L2 L0.end L3.end
  constraint symmetric L2 L11.start L15.start
  constraint symmetric L2 L11.end L15.end
  constraint symmetric L2 L12.start L16.start
  constraint symmetric L2 L12.end L16.end
  constraint symmetric L2 S97.start S101.start
  constraint symmetric L2 S97.end S101.end
  constraint symmetric L2 S97 S101
  measures "d11" distance of L7 L8
  measures "d12" distance of L9 L10
extrude "Extrude1" add sketch "Sketch5" against normal blind 2 contours S0 S1 S2 S44 S45 S46 S72 S73 S74 S75 S92 S93 L5 L13 | S2 S29 S94 S95 | S2 S3 S4 S75 S76 S77 L5 L11 | S28 S29 S30 S31 S32 S33 S34 S35 | S42 S43 S44 S90 S91 S92 L13 L15 | S44 S52 S98 S99 | S47 S48 S49 S50 S51 S52 S53 S54 | S4 S15 L0 S96 S97 | S4 S77 L11 S97 | S4 S5 S6 S7 S8 S9 S10 S36 S37 S38 S39 S40 S41 S42 S77 S78 S79 S80 S81 S82 S83 S84 S85 S86 S87 S88 S89 S90 S97 S101 | S11 S12 S13 S14 S15 L0 L1 S16 S17 S18 S19 S20 S21 S22 S23 S24 S25 S26 S27 S55 S56 S57 S58 S59 L3 L4 S60 S61 S62 S63 S64 S65 S66 S67 S68 S69 S70 S71 | S42 S90 L15 S101 | S42 S59 L3 S100 S101 | S33 S35 S48 S49 L7 L8 | S10 S11 S36 S55 L9 L10
extrude "Extrude2" add sketch "Sketch5" along normal blind 10 contours S0 S1 S2 S44 S45 S46 S72 S73 S74 S75 S92 S93 L5 L13 | S2 S3 S4 S75 S76 S77 L5 L11 | S42 S43 S44 S90 S91 S92 L13 L15 | S4 S77 L11 S97 | S4 S5 S6 S7 S8 S9 S10 S36 S37 S38 S39 S40 S41 S42 S77 S78 S79 S80 S81 S82 S83 S84 S85 S86 S87 S88 S89 S90 S97 S101 | S42 S90 L15 S101
extrude "Extrude3" add sketch "Sketch5" along normal blind 5 contours S28 S29 S30 S31 S32 S33 S34 S35 | S47 S48 S49 S50 S51 S52 S53 S54 | S11 S12 S13 S14 S15 L0 L1 S16 S17 S18 S19 S20 S21 S22 S23 S24 S25 S26 S27 S55 S56 S57 S58 S59 L3 L4 S60 S61 S62 S63 S64 S65 S66 S67 S68 S69 S70 S71